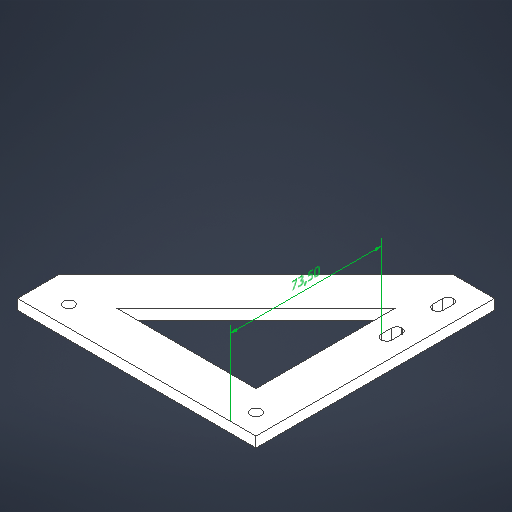
# Autodesk Inventor part: Escuadra soporte motor
Saved by Autodesk Inventor 2026.1 (Build 301233020, 233B)
## iProperties
Created: 2025-11-24
Part Number: Escuadra soporte motor
Material: Generic
Document SubType Name: Modeling
Designer: Tito Luyo Murata
Density: 1 g/cm^3
Appearance: Default
Author: Tito Luyo Murata
Autodesk Inventor part; units mm, degrees
ref_plane "YZ Plane" through (0, 0, 0) normal (1, 0, 0) x (0, 1, 0)
ref_plane "XZ Plane" through (0, 0, 0) normal (0, 1, 0) x (-1, 0, 0)
ref_plane "XY Plane" through (0, 0, 0) normal (0, 0, 1) x (1, 0, 0)
sketch "Sketch1" plane through (0, 0, 0) normal (0, 1, 0) x (-1, 0, 0)
  line L0 (0, 0) -> (0, -116)
  line L1 (0, -116) -> (20, -116)
  line L2 (20, -116) -> (116, -20)
  line L3 (116, -20) -> (116, 0)
  line L4 (116, 0) -> (0, 0)
  circle A0 centre (101, -10) radius 2.6
  circle A1 centre (10, -10) radius 2.6
  line L5 (10.05, -96) -> (9.95, -96)
  line L6 (7.45, -98.5) -> (7.45, -103.5)
  line L7 (9.95, -106) -> (10.05, -106)
  line L8 (12.55, -103.5) -> (12.55, -98.5)
  arc A2 (10.05, -106) -> (12.55, -103.5) centre (10.05, -103.5) ccw
  arc A3 (7.45, -103.5) -> (9.95, -106) centre (9.95, -103.5) ccw
  arc A4 (12.55, -98.5) -> (10.05, -96) centre (10.05, -98.5) ccw
  arc A5 (9.95, -96) -> (7.45, -98.5) centre (9.95, -98.5) ccw
  line L9 (10.05, -71) -> (9.95, -71)
  arc A6 (12.55, -73.5) -> (10.05, -71) centre (10.05, -73.5) ccw
  arc A7 (9.95, -71) -> (7.45, -73.5) centre (9.95, -73.5) ccw
  line L10 (7.45, -73.5) -> (7.45, -78.5)
  line L11 (12.55, -78.5) -> (12.55, -73.5)
  line L12 (9.95, -81) -> (10.05, -81)
  arc A8 (10.05, -81) -> (12.55, -78.5) centre (10.05, -78.5) ccw
  arc A9 (7.45, -78.5) -> (9.95, -81) centre (9.95, -78.5) ccw
  line L13 (87.7157, -20) -> (20, -87.7157)
  line L14 (20, -87.7157) -> (20, -20)
  line L15 (20, -20) -> (87.7157, -20)
  point P0 (10, -96)
  point P1 (10, -106)
  point P2 (10, -71)
  point P3 (10, -81)
  dimension "d0" = 116
  dimension "d1" = 20
  dimension "d2" = 116
  dimension "d3" = 20
  dimension "d4" = 5.2
  dimension "d5" = 10
  dimension "d6" = 15
  dimension "d7" = 5.2
  dimension "d8" = 10
  dimension "d9" = 10
  dimension "d10" = 10
  dimension "d11" = 10
  dimension "d12" = 2.5
  dimension "d13" = 5.1
  dimension "d14" = 2.5
  dimension "d15" = 10
  dimension "d18" = 25
  dimension "d27" = 20
  constraints: 32 end point, 16 point on circle, 10 centre point, 8 tangent, 3 parallel, 3 perpendicular, 2 equal radius, 2 midpoint, 2 vertical, 1 horizontal, 24 other
  measures "d0" distance of L0.start L0.end
  measures "d1" distance of L0.end L1.end
  measures "d2" distance between parallel lines of L0 L3
  measures "d3" distance from line of L2.end L4
  measures "d4" diameter of A0
  measures "d5" distance from line of A0.centre L4
  measures "d6" distance from line of A0.centre L3
  measures "d7" diameter of A1
  measures "d8" distance from line of L4 A1.centre
  measures "d9" distance from line of L0 A1.centre
  measures "d10" distance from line of L0 point (10, -96)
  measures "d11" distance between parallel lines of L1 L7
  measures "d12" radius of A2
  measures "d13" distance between parallel lines of L8 L6
  measures "d14" radius of A4
  measures "d15" vertical distance of point (10, -106) L5.start
  measures "d18" distance of point (10, -96) point (10, -71)
  measures "d27" distance between parallel lines of L2 L13
extrude "Extrusion1" add sketch "Sketch1" along normal blind 5
body "Solid1"
